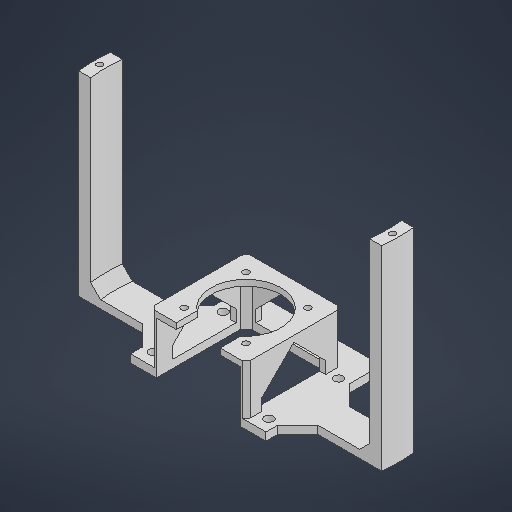
# Autodesk Inventor part: Motor Mount
Saved by Autodesk Inventor 2025.1 (Build 291241000, 241)
## iProperties
Created: 2025-02-24
Part Number: Motor Mount
Material: Generic
Document SubType Name: Modeling
Designer: jerem
Density: 1 g/cm^3
Appearance: Default
Author: jerem
Autodesk Inventor part; units mm, degrees
ref_plane "YZ Plane" through (0, 0, 0) normal (1, 0, 0) x (0, 1, 0)
ref_plane "XZ Plane" through (0, 0, 0) normal (0, 1, 0) x (-1, 0, 0)
ref_plane "XY Plane" through (0, 0, 0) normal (0, 0, 1) x (1, 0, 0)
sketch "Sketch1" plane through (0, 0, 0) normal (0, 1, 0) x (-1, 0, 0)
  line L0 (-21, -21) -> (21, -21)
  line L1 (21, -21) -> (21, 21)
  line L2 (21, 21) -> (-21, 21)
  line L3 (-21, 21) -> (-21, -21)
  line L4 (-21, -21) -> (21, 21) construction
  line L5 (21, -21) -> (-21, 21) construction
  line L6 (-15.5, 15.5) -> (15.5, 15.5) construction
  line L7 (15.5, -15.5) -> (-15.5, -15.5) construction
  line L8 (15.5, 15.5) -> (15.5, -15.5) construction
  circle A0 centre (15.5, 15.5) radius 1.6
  circle A1 centre (15.5, -15.5) radius 1.6
  circle A2 centre (-15.5, -15.5) radius 1.6
  circle A3 centre (-15.5, 15.5) radius 1.6
  line L9 (-24, 24) -> (24, 24)
  line L10 (24, 24) -> (24, -24)
  line L11 (24, -24) -> (-24, -24)
  line L12 (-24, -24) -> (-24, 24)
  line L13 (18, 24) -> (18, 21)
  line L14 (18, 21) -> (21, 18)
  line L15 (21, 18) -> (24, 18)
  line L16 (21, -18) -> (24, -18)
  line L17 (21, -18) -> (18, -21)
  line L18 (18, -21) -> (18, -24)
  line L19 (-18, 24) -> (-18, 21)
  line L20 (-21, 18) -> (-18, 21)
  line L21 (-21, 18) -> (-24, 18)
  line L22 (-24, -18) -> (-21, -18)
  line L23 (-21, -18) -> (-18, -21)
  line L24 (-18, -21) -> (-18, -24)
  circle A4 centre (0, 0) radius 17.5
  line L25 (11, 13.6107) -> (11, 24)
  line L26 (-11, 13.6107) -> (-11, 24)
  line L27 (11, 13.6107) -> (0, 13.6107) construction
  line L28 (0, 13.6107) -> (-11, 13.6107) construction
  line L29 (0, 17.5) -> (0, 13.6107) construction
  line L30 (21, 21) -> (21, 24)
  line L31 (-21, 21) -> (-21, 24)
  line L32 (16, -21) -> (16, -24)
  line L33 (-16, -21) -> (-16, -24)
  line L34 (24, -16) -> (21, -16)
  line L35 (-21, -16) -> (-24, -16)
  line L36 (-21, 16) -> (-24, 16)
  line L37 (24, 16) -> (21, 16)
  dimension "d0" = 42
  dimension "d1" = 42
  dimension "d2" = 31
  dimension "d3" = 3.2
  dimension "d4" = 3
  dimension "d5" = 3
  dimension "d10" = 35
  dimension "d23" = 22
  dimension "d37" = 2
  dimension "d38" = 2
  dimension "d39" = 2
  dimension "d40" = 2
  dimension "d41" = 2
  dimension "d42" = 2
  constraints: 76 end point, 40 point on line, 21 perpendicular, 10 equal length, 5 centre point, 5 coincident, 3 equal radius, 3 point on circle, 2 horizontal, 2 midpoint, 1 vertical, 3 other
  measures "d0" distance of L2.end L1.end
  measures "d1" distance of L1.end L0.end
  measures "d2" distance of L6.end L7.start
  measures "d3" diameter of A0
  measures "d4" distance between parallel lines of L1 L10
  measures "d5" horizontal distance of L1.end L15.end
  measures "d10" diameter of A4
  measures "d23" distance of L26.end L25.end
  measures "d37" distance between parallel lines of L16 L34
  measures "d38" distance between parallel lines of L18 L32
  measures "d39" distance between parallel lines of L24 L33
  measures "d40" distance between parallel lines of L35 L22
  measures "d41" distance between parallel lines of L21 L36
  measures "d42" distance between parallel lines of L15 L37
extrude "Extrusion1" add sketch "Sketch1" along normal blind 3 contours L3 L23 L0 | L0 L24 L11 L12 L22 L3 | L23 L3 L20 L2 L26 A4 L25 L14 L1 L17 L0 | L0 L33 L11 L24 | L22 L12 L35 L3 | L0 L32 L11 L33 | L35 L12 L36 L3 | L0 L18 L11 L32 | L36 L12 L21 L3 | L17 L1 L0 | L0 L1 L16 L10 L11 L18 | L21 L12 L9 L31 L3 | L3 L2 L20 | L1 L34 L10 L16 | L31 L9 L19 L2 | L19 L9 L26 L2 | L1 L37 L10 L34 | L1 L15 L10 L37 | L25 L9 L13 L2 | L14 L2 L1 | L1 L30 L9 L10 L15 | L13 L9 L30 L2
extrude "Extrusion2" add sketch "Sketch1" against normal blind 22 contours L3 L23 L0 | L0 L24 L11 L12 L22 L3 | L0 L33 L11 L24 | L22 L12 L35 L3 | L0 L18 L11 L32 | L36 L12 L21 L3 | L17 L1 L0 | L0 L1 L16 L10 L11 L18 | L21 L12 L9 L31 L3 | L1 L34 L10 L16 | L1 L15 L10 L37 | L1 L30 L9 L10 L15
sketch "Sketch2" plane through (0, -22, 0) normal (0, -1, 0) x (1, 0, 0)
  line L0 (-24, 24) -> (24, 24)
  line L1 (24, 24) -> (24, -24)
  line L2 (24, -24) -> (-24, -24)
  line L3 (-24, -24) -> (-24, 24)
  line L4 (-24, 24) -> (24, -24) construction
  line L5 (24, 24) -> (-24, -24) construction
  line L6 (21, -18) -> (18, -21) projected
  line L7 (16, -24) -> (24, -24) construction
  line L8 (24, -24) -> (24, -16) construction
  line L9 (24, -24) -> (34, -24)
  line L10 (34, -24) -> (34, 24)
  line L11 (34, 24) -> (24, 24)
  line L12 (-24, -24) -> (-34, -24)
  line L13 (-34, -24) -> (-34, 24)
  line L14 (-34, 24) -> (-24, 24)
  circle A0 centre (29, -17.5) radius 2.25
  circle A1 centre (29, 17.5) radius 2.25
  line L15 (29, -17.5) -> (29, 17.5) construction
  line L16 (29, 0) -> (24, 0) construction
  line L17 (-29, -17.5) -> (-29, 17.5) construction
  line L18 (-29, 0) -> (-24, 0) construction
  circle A2 centre (-29, -17.5) radius 2.25
  circle A3 centre (-29, 17.5) radius 2.25
  circle A4 centre (0, 0) radius 70.5
  circle A5 centre (0, 0) radius 76.5
  line L19 (-70.0446, -8) -> (-76.0805, -8)
  line L20 (-70.0446, 8) -> (-76.0805, 8)
  line L21 (-70.0446, -8) -> (-70.0446, 8) construction
  line L22 (-70.0446, 0) -> (-34, 0) construction
  circle A6 centre (-73.5, 0) radius 1.5
  line L23 (-70.5, 0) -> (-73.5, 0) construction
  line L24 (-70.0446, 0) -> (-70.5, 0) construction
  line L25 (-70.0446, -8) -> (-34, -8)
  line L26 (-70.0446, 8) -> (-34, 8)
  line L27 (0, 0) -> (0, 8.579) construction
  line L28 (70.0446, -8) -> (76.0805, -8)
  line L29 (70.0446, 8) -> (76.0805, 8)
  circle A7 centre (73.5, 0) radius 1.5
  line L30 (70.5, 0) -> (73.5, 0) construction
  line L31 (70.0446, 0) -> (70.5, 0) construction
  line L32 (70.0446, -8) -> (34, -8)
  line L33 (70.0446, 8) -> (34, 8)
  line L34 (-24, -24) -> (-16, -24) projected
  line L35 (-16, -24) -> (-16, -21) projected
  line L36 (-16, -21) -> (-18, -21) projected
  line L37 (-18, -21) -> (-21, -18) projected
  line L38 (-21, -18) -> (-21, -16) projected
  line L39 (-21, -16) -> (-24, -16) projected
  line L40 (-24, -16) -> (-24, -24) projected
  line L41 (24, 24) -> (21, 24) projected
  line L42 (21, 24) -> (21, 16) projected
  line L43 (21, 16) -> (24, 16) projected
  line L44 (24, 16) -> (24, 24) projected
  line L45 (18, -21) -> (16, -21) projected
  line L46 (16, -21) -> (16, -24) projected
  line L47 (24, -16) -> (21, -16) projected
  line L48 (21, -16) -> (21, -18) projected
  line L49 (21, -16) -> (21, 16)
  line L50 (16, -21) -> (-16, -21)
  line L51 (-21, -16) -> (-21, 16)
  line L52 (-24, 16) -> (-21, 16) projected
  line L53 (-21, 16) -> (-21, 24) projected
  line L54 (-21, 24) -> (-24, 24) projected
  line L55 (-24, 24) -> (-24, 16) projected
  line L56 (-24, 16) -> (-21, 16) projected
  line L57 (34, -24) -> (34, -34)
  line L58 (34, -34) -> (-34, -34)
  line L59 (-34, -34) -> (-34, -24)
  point P0 (0, 0)
  point P1 (34, 8)
  point P2 (34, -8)
  point P3 (70.0446, -8)
  dimension "d11" = 48
  dimension "d12" = 48
  dimension "d16" = 4.5
  dimension "d17" = 35
  dimension "d18" = 5
  dimension "d19" = 5
  dimension "d24" = 141
  dimension "d25" = 6
  dimension "d26" = 16
  dimension "d27" = 3
  dimension "d28" = 3
  dimension "d46" = 10
  constraints: 74 end point, 13 perpendicular, 9 symmetric about line, 8 centre point, 8 midpoint, 5 coincident, 5 point on circle, 5 point on line, 4 horizontal, 4 vertical, 3 collinear, 3 equal length, 3 equal radius, 3 parallel, 1 other
  measures "d11" distance of L1.end L2.end
  measures "d12" distance of L0.end L1.end
  measures "d16" diameter of A0
  measures "d17" distance of L15.start L15.end
  measures "d18" distance of L16.start L16.end
  measures "d19" distance between parallel lines of L10 L15
  measures "d24" diameter of A4
  measures "d25" radial gap between concentric circles of A4 A5
  measures "d26" distance of L19.start L20.start
  measures "d27" diameter of A6
  measures "d28" distance of L23.start L23.end
  measures "d46" distance between parallel lines of L9 L58
extrude "Extrusion3" add sketch "Sketch2" along normal blind 4 contours L0 L53 L52 L3 | L3 L12 L13 L14 | L52 L51 L39 L3 | L0 L1 L43 L42 | L39 L38 L37 L36 L35 L2 L3 | L13 L25 A4 L26 | L11 L10 L9 L1 | L43 L1 L47 L49 | L2 L9 L57 L58 L59 L12 | A4 L19 A5 L20 | L47 L1 L2 L46 L45 L6 L48 | L35 L50 L46 L2 | L29 A5 L28 A4 | A4 L32 L10 L33
extrude "Extrusion4" add sketch "Sketch2" against normal blind 94 contours A4 L19 A5 L20 | L29 A5 L28 A4
chamfer "Chamfer1" distance 5 angle 45 2 edges at (-70.5, -22, 0) (70.5, -22, 0)
chamfer "Chamfer2" distance 10 angle 45 4 edges at (-34, -24, 8) (-34, -24, -8) (34, -24, 8) (34, -24, -8)
chamfer "Chamfer3" distance 16 angle 45 6 edges at (-22.5, 0, -16) (-22.5, 0, 16) (-16, 0, -22.5) (22.5, 0, 16) (22.5, 0, -16) (16, 0, -22.5)
chamfer "Chamfer4" distance 2 angle 45 4 edges at (-24, -9.5, 24) (24, -9.5, 24) (24, -9.5, -24) (-24, -9.5, -24)
equation "\"d38\" = d37"
equation "\"d39\" = d37"
equation "\"d40\" = d37"
equation "\"d41\" = d37"
equation "\"d42\" = d37"
equation "\"d19\" = d18"
body "Solid1"
